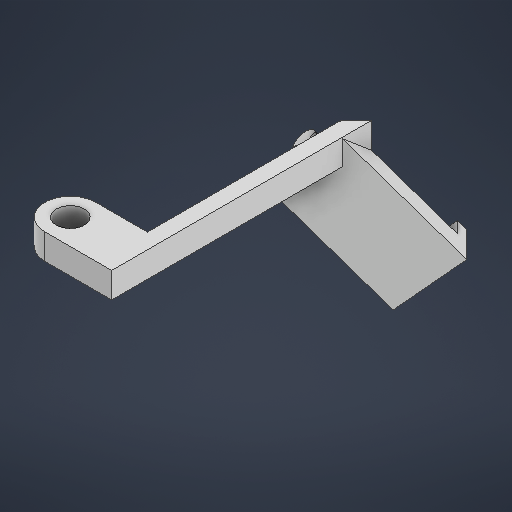
# Autodesk Inventor part: Pixy2 mount
Saved by Autodesk Inventor 2026 (Build 300175050, 175E)
## iProperties
Created: 2025-10-30
Part Number: Pixy2 mount
Material: Generic
Document SubType Name: Modeling
Designer: aduwa
Density: 1 g/cm^3
Appearance: Default
Author: aduwa
Autodesk Inventor part; units mm, degrees
ref_plane "YZ Plane" through (0, 0, 0) normal (1, 0, 0) x (0, 1, 0)
ref_plane "XZ Plane" through (0, 0, 0) normal (0, 1, 0) x (-1, 0, 0)
ref_plane "XY Plane" through (0, 0, 0) normal (0, 0, 1) x (1, 0, 0)
sketch "Sketch2" plane through (0, 0, 0) normal (0, 1, 0) x (-1, 0, 0)
  circle A0 centre (13.1, 80.1) radius 2.75
  circle A1 centre (80.1, 13.1) radius 2.75 construction
  line L0 (13.1, 80.1) -> (13.1, 13.1)
  line L1 (13.1, 13.1) -> (80.1, 13.1)
  line L2 (3, 37.224) -> (37.224, 3)
  line L3 (3, 37.224) -> (51.4, 37.224) construction
  circle A2 centre (80.1, 13.1) radius 2.75
  line L4 (3.1, 112.1) -> (3.1, 79.1)
  line L5 (79.1, 3.1) -> (112.1, 3.1)
  circle A3 centre (13.1, 80.1) radius 5
  line L6 (13.1, 75.1) -> (3, 75.1)
  line L7 (3, 75.1) -> (3, 3)
  line L8 (13.1, 85.1) -> (0, 85.1)
  line L9 (0, 85.1) -> (0, 0)
  circle A4 centre (80.1, 13.1) radius 5
  line L10 (85.1, 13.1) -> (85.1, 0)
  line L11 (75.1, 13.1) -> (75.1, 3)
  line L12 (75.1, 3) -> (3, 3)
  line L13 (85.1, 0) -> (0, 0)
  line L14 (3, 37.224) -> (-4.0711, 30.1529)
  line L15 (3, 37.224) -> (13, 37.224) construction
  point P0 (0, 0)
  point P1 (0, 34.224)
  dimension "d11" = 48.4
  dimension "d12" = 45
  dimension "d13" = 10
  dimension "d14" = 10.1
  dimension "d15" = 13.1
  dimension "d16" = 3
  dimension "d17" = 10
  dimension "d18" = 13.1
  dimension "d19" = 10.1
  dimension "d20" = 10
  dimension "d21" = 135
  constraints: 32 end point, 8 perpendicular, 5 centre point, 4 point on circle, 4 point on line, 4 tangent, 2 coincident, 2 equal length, 2 horizontal, 1 parallel, 1 vertical
  measures "d11" distance of L2.start L2.end
  measures "d12" angle of L2 L3
  measures "d13" diameter of A3
  measures "d14" distance of L6.start L6.end
  measures "d15" distance of L8.start L8.end
  measures "d16" distance between parallel lines of L9 L7
  measures "d17" diameter of A4
  measures "d18" distance of L10.start L10.end
  measures "d19" distance of L11.start L11.end
  measures "d20" distance of L2.start L14.end
  measures "d21" angle of L14 L15
extrude "Extrusion2" add sketch "Sketch2" along normal blind 5 contours L6 L7 L14 L9 L8 A3 | A3
sketch "Sketch4" plane through (-3, 0, 37.224) normal (-0.7071068, 0, -0.7071068) x (-0.7071068, 0, 0.7071068)
  line L0 (0, 0) -> (0, 5) projected
  line L1 (0, 5) -> (-16.134, -14.2277)
  line L2 (0, 5) -> (25.1, 5) construction
  line L3 (-5.9456, -22.7768) -> (10.1884, -3.5491)
  line L4 (10.1884, -3.5491) -> (0, 5)
  line L5 (-5.9456, -22.7768) -> (-16.134, -14.2277)
  point P0 (-28.4426, 0)
  dimension "d33" = 130
  dimension "d34" = 25.1
  dimension "d35" = 13.3
  dimension "d37" = 25.1
  constraints: 10 end point, 2 perpendicular, 1 equal length, 1 horizontal
  measures "d33" angle of L1 L2
  measures "d34" distance of L0.end L1.end
  measures "d35" distance of L1.end L3.start
  measures "d37" distance of L3.start L3.end
extrude "Extrusion3" add sketch "Sketch4" against normal blind 4
sketch "Sketch6" plane through (0, -0.0562, 34.224) normal (-0.7071068, 0, -0.7071068) x (-0.7071068, 0, 0.7071068)
  line L0 (0, 5.0562) -> (4.2426, 5.0562) projected
  line L1 (0, 0.0562) -> (0, 5.0562) projected
  line L2 (0.0471, 0.0562) -> (-11.8913, -14.1715) projected
  line L3 (-11.8913, -14.1715) -> (-1.7029, -22.7206) projected
  line L4 (-1.7029, -22.7206) -> (14.431, -3.4929) projected
  line L5 (14.431, -3.4929) -> (4.2426, 5.0562) projected
  circle A0 centre (6.1229, -3.0486) radius 2.6
  line L6 (4.6432, 4.72) -> (14.755, -3.7647)
  circle A1 centre (-1.5906, -12.2411) radius 2.6
  line L7 (0, 0.0562) -> (0.0471, 0.0562) projected
  line L8 (14.431, -3.4929) -> (4.2426, 5.0562) projected
  line L9 (-6.7971, -18.4461) -> (10.7436, 2.4582)
  point P0 (-24.2, 0.0562)
  dimension "d38" = 5.2
  dimension "d39" = 5
  dimension "d40" = 12
  constraints: 4 end point, 2 centre point, 2 point on line, 1 collinear, 1 equal radius, 1 midpoint, 1 perpendicular
  measures "d38" diameter of A0
  measures "d39" distance from line of L6 A0.centre
  measures "d40" distance of A1.centre A0.centre
extrude "Extrusion5" [suppressed]
fillet "Fillet1" [suppressed]
sketch "Sketch9" plane through (-0.1716, 0, 40.0524) normal (0.7071068, 0, 0.7071068) x (0.7071068, 0, -0.7071068)
  line L0 (4.1955, 0) -> (16.134, -14.2277) projected
  line L1 (16.134, -14.2277) -> (6.4922, -2.737)
  line L2 (6.4922, -2.737) -> (8.7903, -0.8087)
  line L3 (8.7903, -0.8087) -> (18.4321, -12.2994)
  line L4 (18.4321, -12.2994) -> (16.134, -14.2277)
  line L5 (5.9456, -22.7768) -> (16.134, -14.2277) projected
  line L6 (11.0398, -18.5023) -> (9.8066, -17.0326)
  line L7 (5.9456, -22.7768) -> (-3.6962, -11.2861)
  line L8 (-5.9944, -13.2145) -> (3.6474, -24.7052)
  line L9 (-3.6962, -11.2861) -> (-5.9944, -13.2145)
  line L10 (3.6474, -24.7052) -> (5.9456, -22.7768)
  point P0 (28.4426, 0)
  point P1 (4.6202, -0.5061)
  dimension "d46" = 15
  dimension "d47" = 3
  constraints: 18 end point, 4 perpendicular, 3 symmetric about line, 1 midpoint, 1 point on line
  measures "d46" distance of L0.end L1.end
  measures "d47" distance of L1.end L2.end
extrude "Extrusion6" [suppressed]
sketch "Sketch10" plane through (8.4084, -14.2277, 25.8155) normal (0.4545195, -0.7660444, -0.4545195) x (0.7071068, 0, 0.7071068)
  line L0 (0, 0) -> (0, 13.3) projected
  line L1 (0, 0) -> (4, 0) projected
  line L2 (4, 13.3) -> (4, 0) projected
  line L3 (0, 13.3) -> (4, 13.3) projected
  line L4 (-0.6, 8.15) -> (0, 8.15)
  line L5 (0, -1.85) -> (0, 5.15)
  line L6 (0, 5.15) -> (-0.6, 5.15)
  arc A0 (-0.6, 5.15) -> (-1.099, 4.6815) centre (-0.6, 4.65) ccw
  arc A1 (-1.7225, 4.2287) -> (-1.099, 4.6815) centre (-1.598, 4.713) ccw
  arc A2 (-1.7225, 9.0713) -> (-1.7225, 4.2287) centre (-1.1, 6.65) ccw
  arc A3 (-1.099, 8.6185) -> (-1.7225, 9.0713) centre (-1.598, 8.587) ccw
  arc A4 (-1.099, 8.6185) -> (-0.6, 8.15) centre (-0.6, 8.65) ccw
  line L7 (0, 0) -> (0, 13.3) projected
  line L8 (0.6, 5.35) -> (-0.6, 5.35)
  arc A5 (-0.6, 5.35) -> (-1.2986, 4.6941) centre (-0.6, 4.65) ccw
  arc A6 (-1.6727, 4.4224) -> (-1.2986, 4.6941) centre (-1.598, 4.713) ccw
  arc A7 (-1.6727, 8.8776) -> (-1.6727, 4.4224) centre (-1.1, 6.65) ccw
  arc A8 (-1.2986, 8.6059) -> (-1.6727, 8.8776) centre (-1.598, 8.587) ccw
  arc A9 (-1.2986, 8.6059) -> (-0.6, 7.95) centre (-0.6, 8.65) ccw
  line L9 (-0.6, 7.95) -> (0.6, 7.95)
  line L10 (0.3, -1.85) -> (0.3, 5.45)
  line L11 (0.3, 5.45) -> (-0.6, 5.45)
  arc A10 (-0.6, 5.45) -> (-1.3984, 4.7004) centre (-0.6, 4.65) ccw
  arc A11 (-1.6478, 4.5193) -> (-1.3984, 4.7004) centre (-1.598, 4.713) ccw
  arc A12 (-1.6478, 8.7807) -> (-1.6478, 4.5193) centre (-1.1, 6.65) ccw
  arc A13 (-1.3984, 8.5996) -> (-1.6478, 8.7807) centre (-1.598, 8.587) ccw
  arc A14 (-1.3984, 8.5996) -> (-0.6, 7.85) centre (-0.6, 8.65) ccw
  line L12 (-0.6, 7.85) -> (0.4, 7.85)
  line L13 (0.4, -1.85) -> (0.4, 5.55)
  line L14 (0.4, 5.55) -> (-0.6, 5.55)
  arc A15 (-0.6, 5.55) -> (-1.4982, 4.7067) centre (-0.6, 4.65) ccw
  arc A16 (-1.6229, 4.6161) -> (-1.4982, 4.7067) centre (-1.598, 4.713) ccw
  arc A17 (-1.6229, 8.6839) -> (-1.6229, 4.6161) centre (-1.1, 6.65) ccw
  arc A18 (-1.4982, 8.5933) -> (-1.6229, 8.6839) centre (-1.598, 8.587) ccw
  arc A19 (-1.4982, 8.5933) -> (-0.6, 7.75) centre (-0.6, 8.65) ccw
  line L15 (-0.6, 7.75) -> (0.4, 7.75)
  point P0 (-24.2, -18.5744)
  point P1 (-11.4165, -11.1867)
  point P2 (0, 6.65)
  point P3 (0, 6.65)
  point P4 (0, 5.35)
  point P5 (0, 7.95)
  point P6 (0, 5.45)
  point P7 (0, 7.85)
  point P8 (0, 5.55)
  point P9 (0, 7.75)
  dimension "d64" = 2.5
  dimension "d65" = 0.6
  dimension "d66" = 1.1
  dimension "d67" = 0.2
  dimension "d68" = 0.3
  dimension "d69" = 0.4
  constraints: 40 point on circle, 22 end point, 20 centre point, 2 midpoint, 1 collinear, 1 horizontal alignment, 1 parallel, 20 other
  measures "d64" radius of A2
  measures "d65" distance of L5.end L6.end
  measures "d66" distance from line of L5 A2.centre
  measures "d67" radial gap between concentric circles of A2 A7
  measures "d68" radial gap between concentric circles of A2 A12
  measures "d69" radial gap between concentric circles of A2 A17
extrude "Extrusion7" add sketch "Sketch10" against normal up to surface (25.1 mm away) contours L14 A15 A16 A17 A18 A19 L15 L0
sketch "Sketch11" plane through (11.2369, -14.2277, 28.644) normal (0.4545195, -0.7660444, -0.4545195) x (0.7071068, 0, 0.7071068)
  line L0 (-4, 0) -> (-4, 5.55) projected
  line L1 (-4, 0) -> (0, 0) projected
  line L2 (0, 13.3) -> (0, 0) projected
  line L3 (-4, 13.3) -> (0, 13.3) projected
  line L4 (0, 0) -> (0, 13.3)
  line L5 (0, 0) -> (-7.3, 0)
  line L6 (-7.7, 13.3) -> (0, 13.3)
  line L7 (0, 13.3) -> (0, 0)
  line L8 (-4, 7.75) -> (-4, 13.3) projected
  line L9 (-4, 7.75) -> (-4.6, 7.75) projected
  arc A0 (-5.4982, 8.5933) -> (-4.6, 7.75) centre (-4.6, 8.65) ccw projected
  arc A1 (-5.4982, 8.5933) -> (-5.6229, 8.6839) centre (-5.598, 8.587) ccw projected
  arc A2 (-5.6229, 8.6839) -> (-5.6229, 4.6161) centre (-5.1, 6.65) ccw projected
  arc A3 (-5.6229, 4.6161) -> (-5.4982, 4.7067) centre (-5.598, 4.713) ccw projected
  arc A4 (-4.6, 5.55) -> (-5.4982, 4.7067) centre (-4.6, 4.65) ccw projected
  line L10 (-4.6, 5.55) -> (-4, 5.55) projected
  line L11 (-7.2, 13.3) -> (-7.2, 0)
  arc A5 (-5.6229, 8.6839) -> (-5.6229, 4.6161) centre (-5.1, 6.65) ccw projected
  point P0 (-28.2, -18.5744)
  point P1 (-4, 0)
  point P2 (0, 13.3)
  point P3 (0, 0)
  point P4 (-4, 13.3)
  point P5 (-4, 13.3)
  point P6 (-4, 0)
  point P7 (-7.2, 6.65)
  point P8 (-7.2, 6.65)
  constraints: 10 end point, 1 horizontal, 1 midpoint, 1 parallel, 1 perpendicular, 1 point on circle, 1 point on line, 1 tangent
extrude "Extrusion8" add sketch "Sketch11" along normal blind 2
body "Solid2"
